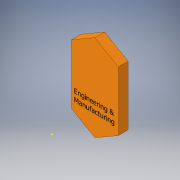
# Autodesk Inventor part: Academies logo
Saved by Autodesk Inventor 2018 (Build 220112000, 112)
## iProperties
Created: 2017-11-06
Part Number: Academies logo
Material: Generic
Document SubType Name: Modeling
Designer: 990813
Density: 1 g/cm^3
Appearance: Orange
Author: 990813
Autodesk Inventor part; units mm, degrees
ref_plane "YZ Plane" through (0, 0, 0) normal (1, 0, 0) x (0, 1, 0)
ref_plane "XZ Plane" through (0, 0, 0) normal (0, 1, 0) x (-1, 0, 0)
ref_plane "XY Plane" through (0, 0, 0) normal (0, 0, 1) x (1, 0, 0)
sketch "Sketch1" plane through (0, 0, 0) normal (0, 0, 1) x (1, 0, 0)
  line L0 (21.6079, 10.4672) -> (13.9879, 6.0678)
  line L1 (13.9879, 6.0678) -> (6.3679, 10.4672)
  line L2 (6.3679, 29.8109) -> (13.9879, 34.2103)
  line L3 (13.9879, 34.2103) -> (21.6079, 29.8109)
  line L4 (6.3679, 29.8109) -> (6.3679, 10.4672)
  line L5 (21.6079, 29.8109) -> (21.6079, 10.4672)
  point P0 (0, 0)
  point P1 (13.9879, 20.1391)
  dimension "d2" = 28.1426
  dimension "d3" = 15.24
  constraints: 12 end point, 1 vertical, 3 other
  measures "d2" distance of L0.end L2.end
  measures "d3" distance between parallel lines of L5 L4
extrude "Extrusion1" add sketch "Sketch1" along normal blind 3.175
sketch "Sketch2" plane through (0, 0, 3.175) normal (0, 0, 1) x (1, 0, 0)
  line L0 (7.1627, 16.7783) -> (25.4618, 16.7783) construction
  line L1 (25.4618, 16.7783) -> (25.4618, 11.2346) construction
  line L2 (25.4618, 11.2346) -> (7.1627, 11.2346) construction
  line L3 (7.1627, 11.2346) -> (7.1627, 16.7783) construction
  point P0 (0, 0)
  constraints: 2 other
body "Solid1"
